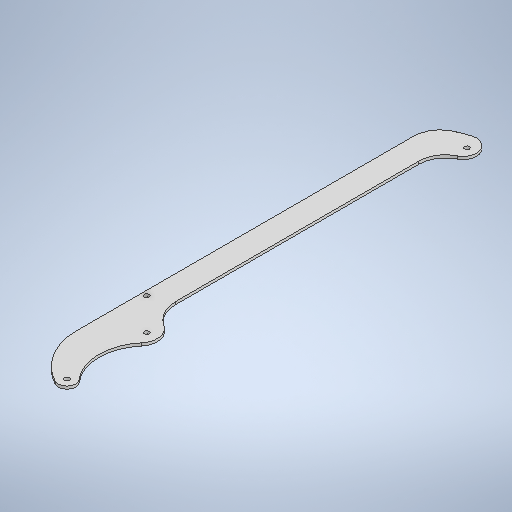
# Autodesk Inventor part: A1P3
Saved by Autodesk Inventor 2025.2 (Build 292293000, 293)
## iProperties
Created: 2025-05-22
Part Number: A1P3
Material: Generic
Document SubType Name: Sheet Metal
Designer: Admin
Density: 1 g/cm^3
Sheet Metal Rule: Default
Appearance: Default
Author: Admin
Autodesk Inventor part; units mm, degrees
ref_plane "YZ Plane" through (0, 0, 0) normal (1, 0, 0) x (0, 1, 0)
ref_plane "XZ Plane" through (0, 0, 0) normal (0, 1, 0) x (-1, 0, 0)
ref_plane "XY Plane" through (0, 0, 0) normal (0, 0, 1) x (1, 0, 0)
sketch "Sketch1" plane through (0, 0, 0) normal (0, 1, 0) x (-1, 0, 0)
  arc A0 (2.5327, 4.8257) -> (-3.8403, -3.8671) centre (0, 0) ccw
  arc A1 (-3.7904, -42.8745) -> (-3.8403, -3.8671) centre (-26.7044, -23.4001) ccw
  line L0 (23.0936, -29.186) -> (23.0936, -239.4885)
  arc A2 (23.0936, -29.186) -> (2.5327, 4.8257) centre (-15.3179, -29.186) ccw
  arc A3 (-3.7904, -42.8745) -> (-1.2456, -59.3257) centre (4.5937, -50) ccw
  line L1 (7.9735, -75.9754) -> (7.9735, -227.7453)
  arc A4 (7.9735, -75.9754) -> (-1.2456, -59.3257) centre (-11.6706, -75.9754) ccw
  arc A5 (-1.1845, -242.5454) -> (7.9735, -227.7453) centre (-8.5646, -227.7453) ccw
  arc A6 (-1.1845, -242.5454) -> (5.4061, -257.8187) centre (2.5327, -250) ccw
  line L2 (5.4061, -257.8187) -> (11.9895, -255.3993)
  arc A7 (11.9895, -255.3993) -> (23.0936, -239.4885) centre (6.1424, -239.4885) ccw
  dimension "d0" = 10.9
  dimension "d1" = 50
  dimension "d4" = 200
  constraints: 16 point on circle, 10 tangent, 8 centre point, 6 end point, 2 vertical, 1 coincident
  measures "d0" diameter of A0
  measures "d1" vertical distance of A3.centre point (0, 0)
  measures "d4" vertical distance of A6.centre A3.centre
extrude "Extrusion1" add sketch "Sketch1" along normal blind 1.7
sketch "Sketch2" plane through (0, 1.7, 0) normal (0, 1, 0) x (1, 0, 0)
  arc A0 (1.1845, 242.5454) -> (-5.4061, 257.8187) centre (-2.5327, 250) ccw projected
  arc A1 (3.7904, 42.8745) -> (1.2456, 59.3257) centre (-4.5937, 50) ccw projected
  arc A2 (-2.5327, -4.8257) -> (3.8403, 3.8671) centre (0, 0) ccw projected
  circle A3 centre (0, 0) radius 1.5
  circle A4 centre (-0.1041, 50) radius 1.5
  circle A5 centre (-20.1041, 70) radius 1.5
  circle A6 centre (-0.1041, 250) radius 1.5
  dimension "d7" = 3
  dimension "d8" = 3
  dimension "d9" = 20
  dimension "d10" = 20
  dimension "d11" = 3
  dimension "d12" = 3
  constraints: 4 centre point, 1 coincident
  measures "d7" diameter of A3
  measures "d8" diameter of A4
  measures "d9" horizontal distance of A5.centre A4.centre
  measures "d10" horizontal distance of A4.centre A5.centre
  measures "d11" diameter of A5
  measures "d12" diameter of A6
extrude "Extrusion2" cut sketch "Sketch2" against normal blind 1.7
equation "\"BendRadius\" = Thickness"
equation "\"BendReliefWidth\" = Thickness"
equation "\"BendReliefDepth\" = 0.5 * Thickness"
equation "\"CornerReliefSize\" = 4 * Thickness"
equation "\"MinimumRemnant\" = 2 * Thickness"
equation "\"TransitionRadius\" = BendRadius"
equation "\"JacobiRadiusSize\" = BendRadius"
equation "\"GapSize\" = Thickness"
equation "\"Thickness\" = 3.048"
body "Solid1"
